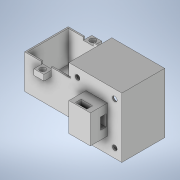
# Autodesk Inventor part: shell 3.0
Saved by Autodesk Inventor 2020.2 (Build 242310000, 310)
## iProperties
Created: 2020-02-10
Part Number: shell 3.0
Material: Generic
Document SubType Name: Modeling
Designer: ColinP
Density: 1 g/cm^3
Appearance: Default
Author: ColinP
Autodesk Inventor part; units mm, degrees
ref_plane "YZ Plane" through (0, 0, 0) normal (1, 0, 0) x (0, 1, 0)
ref_plane "XZ Plane" through (0, 0, 0) normal (0, 1, 0) x (-1, 0, 0)
ref_plane "XY Plane" through (0, 0, 0) normal (0, 0, 1) x (1, 0, 0)
sketch "Sketch1" plane through (0, 0, 0) normal (0, 1, 0) x (-1, 0, 0)
  line L0 (9.0944, 11.3049) -> (-22.9063, 11.3049)
  line L1 (9.0944, 11.3049) -> (41.0951, 11.3049) construction
  line L2 (-22.9063, 11.3049) -> (-22.9063, -19.1751)
  line L3 (-22.9063, -19.1751) -> (9.0944, -19.1751)
  line L4 (9.0944, -19.1751) -> (9.0944, 11.3049)
  point P0 (0, 0)
  dimension "d0" = 32.0007
  dimension "d1" = 180
  dimension "d2" = 30.48
  constraints: 10 end point, 2 horizontal, 2 perpendicular, 1 collinear, 1 vertical
  measures "d0" distance of L0.start L0.end
  measures "d1" angle of L0 L1
  measures "d2" distance of L0.end L2.end
extrude "Extrusion1" add sketch "Sketch1" along normal blind 2
sketch "Sketch2" plane through (0, 2, 0) normal (0, 1, 0) x (1, 0, 0)
  line L0 (-9.0944, 19.1751) -> (-9.0944, -11.3049) projected
  line L1 (-9.0944, -11.3049) -> (-9.0944, -10.3049)
  line L2 (-9.0944, -10.3049) -> (-8.0944, -10.3049)
  line L3 (-9.0944, 19.1751) -> (-8.0944, 19.1751)
  line L4 (22.9063, 19.1751) -> (-9.0944, 19.1751) projected
  line L5 (-8.0944, 19.1751) -> (-8.0944, 18.1751)
  line L6 (22.9063, 19.1751) -> (21.9063, 19.1751)
  line L7 (21.9063, 19.1751) -> (21.9063, 18.1751)
  line L8 (22.9063, -11.3049) -> (22.9063, 19.1751) projected
  line L9 (22.9063, -11.3049) -> (22.9063, -10.3049)
  line L10 (21.9063, -10.3049) -> (22.9063, -10.3049)
  line L11 (-8.0944, -10.3049) -> (21.9063, -10.3049)
  line L12 (21.9063, -10.3049) -> (21.9063, 18.1751)
  line L13 (21.9063, 18.1751) -> (-8.0944, 18.1751)
  line L14 (-8.0944, 18.1751) -> (-8.0944, -10.3049)
  line L15 (-9.0944, -11.3049) -> (22.9063, -11.3049) projected
  line L16 (22.9063, -11.3049) -> (22.9063, 19.1751) projected
  line L17 (22.9063, 19.1751) -> (-9.0944, 19.1751) projected
  line L18 (-9.0944, 19.1751) -> (-9.0944, -11.3049) projected
  line L19 (22.9063, -11.3049) -> (22.9063, -3.3649)
  line L20 (22.9063, 19.1751) -> (22.9063, 11.2351)
  line L21 (22.9063, -3.3649) -> (21.9063, -3.3649)
  line L22 (22.9063, 11.2351) -> (21.9063, 11.2351)
  point P0 (0, 0)
  point P1 (22.9063, -3.3649)
  point P2 (22.9063, 11.2351)
  dimension "d5" = 1
  dimension "d6" = 1
  dimension "d7" = 1
  dimension "d8" = 1
  dimension "d11" = 7.94
  dimension "d12" = 7.94
  constraints: 32 end point, 8 point on line, 6 perpendicular, 2 parallel, 1 horizontal, 1 vertical
  measures "d5" distance of L0.end L1.end
  measures "d6" distance of L1.end L2.end
  measures "d7" distance of L3.end L5.end
  measures "d8" distance of L4.start L6.end
  measures "d11" distance of L15.end L19.end
  measures "d12" distance of L16.end L20.end
extrude "Extrusion3" add sketch "Sketch2" along normal blind 20 contours L3 L5 L14 L2 L0 | L2 L11 L10 L8 L15 L0 | L4 L7 L13 L5 | L4 L8 L22 L12 L7 | L12 L21 L8 L10
sketch "Sketch3" plane through (0, 2, 0) normal (0, 1, 0) x (1, 0, 0)
  line L0 (21.9063, -10.3049) -> (21.9063, -3.3649) projected
  line L1 (22.9063, 11.2351) -> (21.9063, 11.2351) projected
  line L2 (21.9063, -3.3649) -> (21.9063, 11.2351)
  line L3 (21.9063, 11.2351) -> (22.9063, 11.2351)
  line L4 (22.9063, -3.3649) -> (22.9063, 11.2351) projected
  line L5 (22.9063, 11.2351) -> (22.9063, -3.3649)
  line L6 (22.9063, -3.3649) -> (21.9063, -3.3649)
  point P0 (0, 0)
  constraints: 8 end point, 3 perpendicular, 1 vertical
extrude "Extrusion4" add sketch "Sketch3" along normal blind 2
sketch "Sketch4" plane through (0, 22, 0) normal (0, 1, 0) x (1, 0, 0)
  line L0 (22.9063, -11.3049) -> (22.9063, 19.1751) projected
  line L1 (22.9063, 3.9351) -> (5.9063, 3.9351)
  line L2 (5.9063, 3.9351) -> (5.9063, 21.4351)
  line L3 (5.9063, 21.4351) -> (5.9063, -13.5649)
  circle A0 centre (5.9063, -13.5649) radius 2
  circle A1 centre (5.9063, 21.4351) radius 2
  line L4 (22.9063, 19.1751) -> (-9.0944, 19.1751) projected
  line L5 (5.9063, 19.1751) -> (2.4063, 19.1751)
  line L6 (2.4063, 19.1751) -> (2.4063, 24.1751)
  line L7 (2.4063, 24.1751) -> (9.4063, 24.1751)
  line L8 (9.4063, 24.1751) -> (9.4063, 19.1751)
  line L9 (9.4063, -11.3049) -> (9.4063, -16.3049)
  line L10 (9.4063, -16.3049) -> (2.4063, -16.3049)
  line L11 (2.4063, -16.3049) -> (2.4063, -11.3049)
  line L12 (-9.0944, -11.3049) -> (22.9063, -11.3049) projected
  point P0 (0, 0)
  dimension "d17" = 17
  dimension "d18" = 17.5
  dimension "d19" = 35
  dimension "d20" = 4
  dimension "d21" = 4
  dimension "d22" = 3.5
  dimension "d23" = 5
  dimension "d24" = 7
  dimension "d25" = 5
  constraints: 20 end point, 10 point on line, 5 perpendicular, 2 centre point, 2 coincident, 1 horizontal, 1 midpoint
  measures "d17" distance of L1.start L1.end
  measures "d18" distance of L1.end L2.end
  measures "d19" distance of L2.end L3.end
  measures "d20" diameter of A0
  measures "d21" diameter of A1
  measures "d22" distance of L5.start L5.end
  measures "d23" distance of L5.end L6.end
  measures "d24" distance of L6.end L7.end
  measures "d25" distance of L9.start L9.end
extrude "Extrusion5" add sketch "Sketch4" against normal blind 4 contours L9 L10 L11 L12 | L4 L6 L7 L8
sketch "Sketch5" plane through (0, 22, 0) normal (0, 1, 0) x (1, 0, 0)
  line L0 (2.4063, 19.1751) -> (2.4063, 24.1751) projected
  line L1 (2.4063, 19.1751) -> (2.4063, 18.1751)
  line L2 (-8.0944, 18.1751) -> (21.9063, 18.1751) projected
  line L3 (22.9063, 19.1751) -> (9.4063, 19.1751) projected
  line L4 (9.4063, 19.1751) -> (9.4063, 18.1751)
  line L5 (-9.0944, -11.3049) -> (22.9063, -11.3049) projected
  line L6 (2.4063, -11.3049) -> (2.4063, -10.3049)
  line L7 (-8.0944, -10.3049) -> (21.9063, -10.3049) projected
  line L8 (9.4063, -10.3049) -> (9.4063, -11.3049)
  circle A0 centre (5.9063, 21.4351) radius 2 projected
  circle A1 centre (5.9063, -13.5649) radius 2 projected
  line L9 (21.9063, -10.3049) -> (-8.0944, -10.3049) projected
  line L10 (-8.0944, -10.3049) -> (-8.0944, 18.1751) projected
  line L11 (-8.0944, 18.1751) -> (21.9063, 18.1751) projected
  line L12 (21.9063, 18.1751) -> (21.9063, 11.2351) projected
  line L13 (21.9063, 11.2351) -> (22.9063, 11.2351) projected
  line L14 (22.9063, 11.2351) -> (22.9063, 19.1751) projected
  line L15 (22.9063, 19.1751) -> (9.4063, 19.1751) projected
  line L16 (9.4063, 19.1751) -> (9.4063, 24.1751) projected
  line L17 (9.4063, 24.1751) -> (2.4063, 24.1751) projected
  line L18 (2.4063, 24.1751) -> (2.4063, 19.1751) projected
  line L19 (2.4063, 19.1751) -> (-9.0944, 19.1751) projected
  line L20 (-9.0944, 19.1751) -> (-9.0944, -11.3049) projected
  line L21 (-9.0944, -11.3049) -> (2.4063, -11.3049) projected
  line L22 (2.4063, -11.3049) -> (2.4063, -16.3049) projected
  line L23 (2.4063, -16.3049) -> (9.4063, -16.3049) projected
  line L24 (9.4063, -16.3049) -> (9.4063, -11.3049) projected
  line L25 (9.4063, -11.3049) -> (22.9063, -11.3049) projected
  line L26 (22.9063, -11.3049) -> (22.9063, -3.3649) projected
  line L27 (22.9063, -3.3649) -> (21.9063, -3.3649) projected
  line L28 (21.9063, -3.3649) -> (21.9063, -10.3049) projected
  point P0 (0, 0)
  point P1 (-8.0944, 18.1751)
  point P2 (22.9063, 19.1751)
  constraints: 8 end point, 4 point on line, 3 vertical, 1 perpendicular
extrude "Extrusion6" add sketch "Sketch5" along normal blind 2 contours L1 L2 L10 L7 L6 L5 L20 L19 | L4 L3 L14 L13 L12 L2 | L8 L7 L28 L27 L26 L5
sketch "Sketch35" plane through (-9.0944, 0, 11.3049) normal (0, 0, 1) x (1, 0, 0)
  line L0 (32.0007, 0) -> (32.0007, 24) projected
  line L1 (32.0007, 12) -> (32.0007, 32)
  line L2 (32.0007, 32) -> (67.0007, 32)
  line L3 (67.0007, 32) -> (67.0007, -8)
  line L4 (67.0007, -8) -> (32.0007, -8)
  line L5 (32.0007, -8) -> (32.0007, 0)
  point P0 (9.0944, 0)
  dimension "d177" = 20
  dimension "d178" = 35
  dimension "d179" = 40
  constraints: 10 end point, 3 perpendicular, 1 midpoint, 1 point on line, 1 vertical
  measures "d177" distance of L1.start L1.end
  measures "d178" distance of L1.end L2.end
  measures "d179" distance of L2.end L3.end
extrude "Extrusion32" add sketch "Sketch35" against normal blind 1
sketch "Sketch36" plane through (-9.0944, 0, 10.3049) normal (0, 0, -1) x (-1, 0, 0)
  line L0 (-32.0007, 32) -> (-32.0007, 24) projected
  line L1 (-32.0007, 32) -> (-37.0007, 32)
  line L2 (-32.0007, 32) -> (-67.0007, 32) projected
  line L3 (-37.0007, 32) -> (-37.0007, 27)
  line L4 (-37.0007, 27) -> (-37.0007, -2.6)
  line L5 (-37.0007, -2.6) -> (-63.0507, -2.6)
  line L6 (-63.0507, -2.6) -> (-63.0507, 27)
  point P0 (-9.0944, 0)
  dimension "d182" = 5
  dimension "d183" = 5
  dimension "d184" = 29.6
  dimension "d185" = 26.05
  dimension "d186" = 29.6
  dimension "d187" = 90
  constraints: 10 end point, 3 perpendicular, 2 point on line
  measures "d182" distance of L0.start L1.end
  measures "d183" distance of L1.end L3.end
  measures "d184" distance of L3.end L4.end
  measures "d185" distance of L4.end L5.end
  measures "d186" distance of L5.end L6.end
  measures "d187" angle of L5 L6
hole "Hole3" at (27.9063, 27, 10.3049) at (53.9563, 27, 10.3049) at (53.9563, -2.6, 10.3049) at (27.9063, -2.6, 10.3049) direction (0, 0, 1) diameter 3.4 end through all
sketch "Sketch37" plane through (-9.0944, 0, 10.3049) normal (0, 0, -1) x (-1, 0, 0)
  point P0 (-9.0944, 0)
sketch "Sketch38" plane through (2.4063, 18, 11.3049) normal (0, 0, 1) x (1, 0, 0)
  line L0 (20.5, -18) -> (20.5, 6) projected
  line L1 (19.5, -16) -> (19.5, 6) projected
  line L2 (20.5, 6) -> (19.5, 6)
  line L3 (19.5, 6) -> (19.5, 15)
  line L4 (19.5, 15) -> (56.5, 15)
  line L5 (56.5, 15) -> (56.5, -27)
  line L6 (56.5, -27) -> (19.5, -27)
  line L7 (19.5, -27) -> (19.5, 15)
  circle A0 centre (51.55, -20.6) radius 1.7 projected
  circle A1 centre (25.5, 9) radius 1.7 projected
  circle A2 centre (51.55, 9) radius 1.7 projected
  circle A3 centre (25.5, -20.6) radius 1.7 projected
  line L8 (0, 0) -> (0, 4) projected
  line L9 (0, 4) -> (0, 6) projected
  line L10 (-11.5007, 6) -> (0, 6) projected
  line L11 (-11.5007, -18) -> (-11.5007, 6) projected
  line L12 (-11.5007, -18) -> (20.5, -18) projected
  line L13 (20.5, -18) -> (20.5, -26) projected
  line L14 (20.5, -26) -> (55.5, -26) projected
  line L15 (55.5, -26) -> (55.5, 14) projected
  line L16 (55.5, 14) -> (20.5, 14) projected
  line L17 (20.5, 14) -> (20.5, 6) projected
  line L18 (7, 6) -> (20.5, 6) projected
  line L19 (7, 4) -> (7, 6) projected
  line L20 (7, 4) -> (7, 0) projected
  line L21 (7, 0) -> (0, 0) projected
  line L22 (20.5, 15) -> (21.5, 15)
  line L23 (21.5, 15) -> (21.5, 6)
  line L24 (20.5, 6) -> (20.5, 14) projected
  line L25 (21.5, 6) -> (20.5, 6)
  line L26 (20.5, -26) -> (21.5, -26)
  line L27 (55.5, -26) -> (20.5, -26) projected
  line L28 (21.5, -26) -> (21.5, -18)
  line L29 (20.5, -18) -> (-11.5007, -18) projected
  line L30 (21.5, -18) -> (20.5, -18)
  line L31 (20.5, -26) -> (20.5, -27)
  line L32 (20.5, 14) -> (20.5, 15)
  line L33 (19.5, -16) -> (19.5, 6) projected
  line L34 (19.5, 6) -> (19.5, 7)
  line L35 (19.5, 7) -> (20.5, 7)
  point P0 (-2.4063, -18)
  point P1 (19.5, 7)
  point P2 (20.5, 7)
  point P3 (19.5, -18)
  dimension "d195" = 1
  dimension "d196" = 9
  dimension "d197" = 37
  dimension "d198" = 42
  dimension "d199" = 1
  dimension "d200" = 1
  dimension "d201" = 1
  constraints: 32 end point, 7 perpendicular, 6 point on line, 3 parallel, 2 horizontal, 1 collinear
  measures "d195" distance of L0.end L1.end
  measures "d196" distance of L1.end L3.end
  measures "d197" distance of L5.end L6.end
  measures "d198" distance of L4.end L5.end
  measures "d199" distance of L22.start L22.end
  measures "d200" distance of L13.end L26.end
  measures "d201" distance of L1.end L34.end
extrude "Extrusion33" add sketch "Sketch38" against normal blind 30 contours L13 L31 L6 L7 L12 | L14 L15 L16 L23 L4 L5 L6 L31 | L35 L3 L4 L32 L17 | L32 L4 L23 L16
sketch "Sketch39" plane through (2.4063, 18, 11.3049) normal (0, 0, 1) x (1, 0, 0)
  line L0 (56.5, 15) -> (56.5, -27) projected
  line L1 (56.5, -6) -> (46.5, -6)
  line L2 (46.5, -6) -> (46.5, 4)
  line L3 (46.5, 4) -> (31.5, 4)
  line L4 (31.5, 4) -> (31.5, -16)
  line L5 (31.5, -16) -> (46.5, -16)
  line L6 (46.5, -16) -> (46.5, -6)
  point P0 (-2.4063, -18)
  dimension "d204" = 10
  dimension "d205" = 10
  dimension "d206" = 15
  dimension "d207" = 90
  dimension "d208" = 20
  dimension "d209" = 90
  constraints: 12 end point, 5 perpendicular, 1 horizontal, 1 midpoint, 1 point on line
  measures "d204" distance of L1.start L1.end
  measures "d205" distance of L1.end L2.end
  measures "d206" distance of L2.end L3.end
  measures "d207" angle of L3 L2
  measures "d208" distance of L3.end L4.end
  measures "d209" angle of L4 L3
extrude "Extrusion34" add sketch "Sketch39" along normal blind 12
sketch "Sketch40" plane through (33.9063, 22, 11.3049) normal (0, 1, 0) x (1, 0, 0)
  line L0 (15, -12) -> (0, -12) projected
  line L1 (0, -12) -> (3.5, -12)
  line L2 (3.5, -12) -> (3.5, -11)
  line L3 (3.5, -11) -> (11.5, -11)
  line L4 (11.5, -11) -> (11.5, -7)
  line L5 (11.5, -7) -> (3.5, -7)
  line L6 (3.5, -7) -> (3.5, -11)
  point P0 (-33.9063, 11.3049)
  dimension "d212" = 3.5
  dimension "d213" = 1
  dimension "d214" = 8
  dimension "d215" = 4
  constraints: 12 end point, 2 parallel, 2 perpendicular, 1 horizontal, 1 point on line
  measures "d212" distance of L0.end L1.end
  measures "d213" distance of L1.end L2.end
  measures "d214" distance of L5.end L4.end
  measures "d215" distance of L4.end L3.end
extrude "Extrusion35" cut sketch "Sketch40" against normal up to next
sketch "Sketch41" plane through (33.9063, 2, 11.3049) normal (-1, 0, 0) x (0, 0, 1)
  line L0 (0, -2) -> (0, 22) projected
  line L1 (0, -0.0141) -> (0, 5.9859)
  line L2 (0, 5.9859) -> (1, 5.9859)
  line L3 (1, 5.9859) -> (5, 5.9859)
  line L4 (5, 5.9859) -> (5, 13.9859)
  line L5 (5, 13.9859) -> (1, 13.9859)
  line L6 (1, 13.9859) -> (1, 5.9859)
  point P0 (-11.3049, -2)
  dimension "d218" = 6
  dimension "d219" = 1
  dimension "d220" = 4
  dimension "d221" = 8
  constraints: 12 end point, 2 parallel, 2 perpendicular, 2 point on line, 1 horizontal
  measures "d218" distance of L1.start L1.end
  measures "d219" distance of L1.end L2.end
  measures "d220" distance of L5.end L4.end
  measures "d221" distance of L4.end L3.end
extrude "Extrusion36" cut sketch "Sketch41" against normal up to next
body "Solid1"
